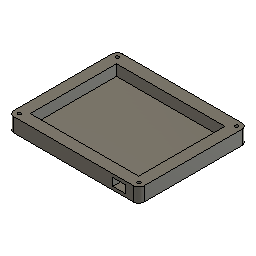
Final assemby 12 key hackpad (Autodesk Fusion 360 archive; units mm, degrees)
design "krish hackpad"
part number: 2026-03-11-19-54-52-839
Autodesk Fusion 360 part; units mm, degrees
sketch "hackpad base" plane through (0, 0, 0) normal (0, 1, 0) x (1, 0, 0)
  line L0 (0, 79.43) -> (0, 0)
  line L1 (0, 0) -> (99.82, 0)
  line L2 (99.82, 0) -> (99.82, 79.43)
  line L3 (99.82, 79.43) -> (0, 79.43)
  line L4 (-10, 90) -> (110, 90)
  line L5 (-10, -10) -> (-10, 90)
  line L6 (110, -10) -> (-10, -10)
  line L7 (110, 90) -> (110, -10)
  circle A0 centre (-5, -5) radius 1.45
  circle A1 centre (105, -5) radius 1.45
  circle A2 centre (105, 85) radius 1.45
  circle A3 centre (-5, 85) radius 1.45
extrude "Extrude1" add sketch "hackpad base" along normal blind 3 contours L0 L1 L2 L3 | L4 L5 L6 L7 makes body 1
extrude "Extrude2" add sketch "hackpad base" along normal blind 13 bodies 1
sketch "yes" plane through (0, 13, 0) normal (0, 1, 0) x (1, 0, 0)
  line L0 (4.775, 74.075) -> (17.775, 74.075)
  line L1 (4.775, 60.075) -> (17.775, 60.075)
  line L2 (4.275, 73.575) -> (4.275, 60.575)
  line L3 (18.275, 73.575) -> (18.275, 60.575)
  arc A0 (4.775, 74.075) -> (4.275, 73.575) centre (4.775, 73.575) ccw
  arc A1 (18.275, 73.575) -> (17.775, 74.075) centre (17.775, 73.575) ccw
  arc A2 (4.275, 60.575) -> (4.775, 60.075) centre (4.775, 60.575) ccw
  arc A3 (17.775, 60.075) -> (18.275, 60.575) centre (17.775, 60.575) ccw
  line L4 (23.825, 74.075) -> (36.825, 74.075)
  line L5 (23.825, 60.075) -> (36.825, 60.075)
  line L6 (23.325, 73.575) -> (23.325, 60.575)
  line L7 (37.325, 73.575) -> (37.325, 60.575)
  arc A4 (23.825, 74.075) -> (23.325, 73.575) centre (23.825, 73.575) ccw
  arc A5 (37.325, 73.575) -> (36.825, 74.075) centre (36.825, 73.575) ccw
  arc A6 (23.325, 60.575) -> (23.825, 60.075) centre (23.825, 60.575) ccw
  arc A7 (36.825, 60.075) -> (37.325, 60.575) centre (36.825, 60.575) ccw
  line L8 (42.875, 74.075) -> (55.875, 74.075)
  line L9 (42.875, 60.075) -> (55.875, 60.075)
  line L10 (42.375, 73.575) -> (42.375, 60.575)
  line L11 (56.375, 73.575) -> (56.375, 60.575)
  arc A8 (42.875, 74.075) -> (42.375, 73.575) centre (42.875, 73.575) ccw
  arc A9 (56.375, 73.575) -> (55.875, 74.075) centre (55.875, 73.575) ccw
  arc A10 (42.375, 60.575) -> (42.875, 60.075) centre (42.875, 60.575) ccw
  arc A11 (55.875, 60.075) -> (56.375, 60.575) centre (55.875, 60.575) ccw
  line L12 (61.925, 74.075) -> (74.925, 74.075)
  line L13 (61.925, 60.075) -> (74.925, 60.075)
  line L14 (61.425, 73.575) -> (61.425, 60.575)
  line L15 (75.425, 73.575) -> (75.425, 60.575)
  arc A12 (61.925, 74.075) -> (61.425, 73.575) centre (61.925, 73.575) ccw
  arc A13 (75.425, 73.575) -> (74.925, 74.075) centre (74.925, 73.575) ccw
  arc A14 (61.425, 60.575) -> (61.925, 60.075) centre (61.925, 60.575) ccw
  arc A15 (74.925, 60.075) -> (75.425, 60.575) centre (74.925, 60.575) ccw
  line L16 (4.775, 55.025) -> (17.775, 55.025)
  line L17 (4.775, 41.025) -> (17.775, 41.025)
  line L18 (4.275, 54.525) -> (4.275, 41.525)
  line L19 (18.275, 54.525) -> (18.275, 41.525)
  arc A16 (4.775, 55.025) -> (4.275, 54.525) centre (4.775, 54.525) ccw
  arc A17 (18.275, 54.525) -> (17.775, 55.025) centre (17.775, 54.525) ccw
  arc A18 (4.275, 41.525) -> (4.775, 41.025) centre (4.775, 41.525) ccw
  arc A19 (17.775, 41.025) -> (18.275, 41.525) centre (17.775, 41.525) ccw
  line L20 (23.825, 55.025) -> (36.825, 55.025)
  line L21 (23.825, 41.025) -> (36.825, 41.025)
  line L22 (23.325, 54.525) -> (23.325, 41.525)
  line L23 (37.325, 54.525) -> (37.325, 41.525)
  arc A20 (23.825, 55.025) -> (23.325, 54.525) centre (23.825, 54.525) ccw
  arc A21 (37.325, 54.525) -> (36.825, 55.025) centre (36.825, 54.525) ccw
  arc A22 (23.325, 41.525) -> (23.825, 41.025) centre (23.825, 41.525) ccw
  arc A23 (36.825, 41.025) -> (37.325, 41.525) centre (36.825, 41.525) ccw
  line L24 (42.875, 55.025) -> (55.875, 55.025)
  line L25 (42.875, 41.025) -> (55.875, 41.025)
  line L26 (42.375, 54.525) -> (42.375, 41.525)
  line L27 (56.375, 54.525) -> (56.375, 41.525)
  arc A24 (42.875, 55.025) -> (42.375, 54.525) centre (42.875, 54.525) ccw
  arc A25 (56.375, 54.525) -> (55.875, 55.025) centre (55.875, 54.525) ccw
  arc A26 (42.375, 41.525) -> (42.875, 41.025) centre (42.875, 41.525) ccw
  arc A27 (55.875, 41.025) -> (56.375, 41.525) centre (55.875, 41.525) ccw
  line L28 (61.925, 55.025) -> (74.925, 55.025)
  line L29 (61.925, 41.025) -> (74.925, 41.025)
  line L30 (61.425, 54.525) -> (61.425, 41.525)
  line L31 (75.425, 54.525) -> (75.425, 41.525)
  arc A28 (61.925, 55.025) -> (61.425, 54.525) centre (61.925, 54.525) ccw
  arc A29 (75.425, 54.525) -> (74.925, 55.025) centre (74.925, 54.525) ccw
  arc A30 (61.425, 41.525) -> (61.925, 41.025) centre (61.925, 41.525) ccw
  arc A31 (74.925, 41.025) -> (75.425, 41.525) centre (74.925, 41.525) ccw
  line L32 (4.775, 35.975) -> (17.775, 35.975)
  line L33 (4.775, 21.975) -> (17.775, 21.975)
  line L34 (4.275, 35.475) -> (4.275, 22.475)
  line L35 (18.275, 35.475) -> (18.275, 22.475)
  arc A32 (4.775, 35.975) -> (4.275, 35.475) centre (4.775, 35.475) ccw
  arc A33 (18.275, 35.475) -> (17.775, 35.975) centre (17.775, 35.475) ccw
  arc A34 (4.275, 22.475) -> (4.775, 21.975) centre (4.775, 22.475) ccw
  arc A35 (17.775, 21.975) -> (18.275, 22.475) centre (17.775, 22.475) ccw
  line L36 (23.825, 35.975) -> (36.825, 35.975)
  line L37 (23.825, 21.975) -> (36.825, 21.975)
  line L38 (23.325, 35.475) -> (23.325, 22.475)
  line L39 (37.325, 35.475) -> (37.325, 22.475)
  arc A36 (23.825, 35.975) -> (23.325, 35.475) centre (23.825, 35.475) ccw
  arc A37 (37.325, 35.475) -> (36.825, 35.975) centre (36.825, 35.475) ccw
  arc A38 (23.325, 22.475) -> (23.825, 21.975) centre (23.825, 22.475) ccw
  arc A39 (36.825, 21.975) -> (37.325, 22.475) centre (36.825, 22.475) ccw
  line L40 (42.875, 35.975) -> (55.875, 35.975)
  line L41 (42.875, 21.975) -> (55.875, 21.975)
  line L42 (42.375, 35.475) -> (42.375, 22.475)
  line L43 (56.375, 35.475) -> (56.375, 22.475)
  arc A40 (42.875, 35.975) -> (42.375, 35.475) centre (42.875, 35.475) ccw
  arc A41 (56.375, 35.475) -> (55.875, 35.975) centre (55.875, 35.475) ccw
  arc A42 (42.375, 22.475) -> (42.875, 21.975) centre (42.875, 22.475) ccw
  arc A43 (55.875, 21.975) -> (56.375, 22.475) centre (55.875, 22.475) ccw
  line L44 (61.925, 35.975) -> (74.925, 35.975)
  line L45 (61.925, 21.975) -> (74.925, 21.975)
  line L46 (61.425, 35.475) -> (61.425, 22.475)
  line L47 (75.425, 35.475) -> (75.425, 22.475)
  arc A44 (61.925, 35.975) -> (61.425, 35.475) centre (61.925, 35.475) ccw
  arc A45 (75.425, 35.475) -> (74.925, 35.975) centre (74.925, 35.475) ccw
  arc A46 (61.425, 22.475) -> (61.925, 21.975) centre (61.925, 22.475) ccw
  arc A47 (74.925, 21.975) -> (75.425, 22.475) centre (74.925, 22.475) ccw
  line L48 (4.775, 16.925) -> (17.775, 16.925)
  line L49 (4.775, 2.925) -> (17.775, 2.925)
  line L50 (4.275, 16.425) -> (4.275, 3.425)
  line L51 (18.275, 16.425) -> (18.275, 3.425)
  arc A48 (4.775, 16.925) -> (4.275, 16.425) centre (4.775, 16.425) ccw
  arc A49 (18.275, 16.425) -> (17.775, 16.925) centre (17.775, 16.425) ccw
  arc A50 (4.275, 3.425) -> (4.775, 2.925) centre (4.775, 3.425) ccw
  arc A51 (17.775, 2.925) -> (18.275, 3.425) centre (17.775, 3.425) ccw
  line L52 (23.825, 16.925) -> (36.825, 16.925)
  line L53 (23.825, 2.925) -> (36.825, 2.925)
  line L54 (23.325, 16.425) -> (23.325, 3.425)
  line L55 (37.325, 16.425) -> (37.325, 3.425)
  arc A52 (23.825, 16.925) -> (23.325, 16.425) centre (23.825, 16.425) ccw
  arc A53 (37.325, 16.425) -> (36.825, 16.925) centre (36.825, 16.425) ccw
  arc A54 (23.325, 3.425) -> (23.825, 2.925) centre (23.825, 3.425) ccw
  arc A55 (36.825, 2.925) -> (37.325, 3.425) centre (36.825, 3.425) ccw
  line L56 (42.875, 16.925) -> (55.875, 16.925)
  line L57 (42.875, 2.925) -> (55.875, 2.925)
  line L58 (42.375, 16.425) -> (42.375, 3.425)
  line L59 (56.375, 16.425) -> (56.375, 3.425)
  arc A56 (42.875, 16.925) -> (42.375, 16.425) centre (42.875, 16.425) ccw
  arc A57 (56.375, 16.425) -> (55.875, 16.925) centre (55.875, 16.425) ccw
  arc A58 (42.375, 3.425) -> (42.875, 2.925) centre (42.875, 3.425) ccw
  arc A59 (55.875, 2.925) -> (56.375, 3.425) centre (55.875, 3.425) ccw
  line L60 (61.925, 16.925) -> (74.925, 16.925)
  line L61 (61.925, 2.925) -> (74.925, 2.925)
  line L62 (61.425, 16.425) -> (61.425, 3.425)
  line L63 (75.425, 16.425) -> (75.425, 3.425)
  arc A60 (61.925, 16.925) -> (61.425, 16.425) centre (61.925, 16.425) ccw
  arc A61 (75.425, 16.425) -> (74.925, 16.925) centre (74.925, 16.425) ccw
  arc A62 (61.425, 3.425) -> (61.925, 2.925) centre (61.925, 3.425) ccw
  arc A63 (74.925, 2.925) -> (75.425, 3.425) centre (74.925, 3.425) ccw
  line L64 (1.75, 0.4) -> (77.95, 0.4)
  line L65 (1.75, 76.6) -> (77.95, 76.6)
  line L66 (1.75, 0.4) -> (1.75, 76.6)
  line L67 (77.95, 0.4) -> (77.95, 76.6)
sketch "Sketch3" plane through (0, 13, 0) normal (0, 1, 0) x (-1, 0, 0)
  circle A0 centre (5, 5) radius 1.45
  line L0 (0, -79.43) -> (-99.82, -79.43)
  line L1 (-99.82, -79.43) -> (-99.82, 0)
  line L2 (-99.82, 0) -> (0, 0)
  line L3 (0, 0) -> (0, -79.43)
  circle A1 centre (-105, 5) radius 1.45
  circle A2 centre (5, -85) radius 1.45
  circle A3 centre (-105, -85) radius 1.45
  line L4 (-110, -90) -> (10, -90)
  line L5 (10, -90) -> (10, 10)
  line L6 (10, 10) -> (-110, 10)
  line L7 (-110, 10) -> (-110, -90)
  line L8 (0, -79.43) -> (-99.82, -79.43)
  line L9 (-99.82, -79.43) -> (-99.82, 0)
  line L10 (-99.82, 0) -> (0, 0)
  line L11 (0, 0) -> (0, -79.43)
  constraint horizontal L8
  constraint vertical L9
  constraint horizontal L10
  constraint vertical L11
  constraint coincident L1.end L2.start
  constraint coincident L0.start L3.end
extrude "Extrude3" add sketch "Sketch3" along normal blind 3 separate body contours L0 L1 L2 L3 L8 L9 L10 L11 | L4 L5 L6 L7 makes body 2
extrude "Extrude4" cut sketch "yes" along normal blind 5 contours L0 L1 L2 L3 A0 A1 A2 A3 | L4 L5 L6 L7 A4 A5 A6 A7 | L8 L9 L10 L11 A8 A9 A10 A11 | L12 L13 L14 L15 A12 A13 A14 A15 | L16 L17 L18 L19 A16 A17 A18 A19 | L20 L21 L22 L23 A20 A21 A22 A23 | L24 L25 L26 L27 A24 A25 A26 A27 | L28 L29 L30 L31 A28 A29 A30 A31 | L32 L33 L34 L35 A32 A33 A34 A35 | L36 L37 L38 L39 A36 A37 A38 A39 | L40 L41 L42 L43 A40 A41 A42 A43 | L44 L45 L46 L47 A44 A45 A46 A47 | L48 L49 L50 L51 A48 A49 A50 A51 | L52 L53 L54 L55 A52 A53 A54 A55 | L56 L57 L58 L59 A56 A57 A58 A59 | L60 L61 L62 L63 A60 A61 A62 A63 bodies 2
fillet "Fillet1" radius 5 8 edges at (-10, 6.5, 10) (-10, 6.5, -90) (110, 6.5, -90) (110, 6.5, 10) (-10, 14.5, 10) (-10, 14.5, -90) (110, 14.5, -90) (110, 14.5, 10) on bodies 1 2
sketch "Sketch4" plane through (0, 16, 0) normal (0, 1, 0) x (-1, 0, 0)
  arc A0 (-105, 10) -> (-110, 5) centre (-105, 5) ccw
  line L0 (-110, 5) -> (-110, -85)
  arc A1 (-110, -85) -> (-105, -90) centre (-105, -85) ccw
  line L1 (-105, -90) -> (5, -90)
  arc A2 (5, -90) -> (10, -85) centre (5, -85) ccw
  line L2 (10, -85) -> (10, 5)
  arc A3 (10, 5) -> (5, 10) centre (5, 5) ccw
  line L3 (5, 10) -> (-105, 10)
  line L4 (-4.775, -35.975) -> (-17.775, -35.975)
  arc A4 (-18.275, -35.475) -> (-17.775, -35.975) centre (-17.775, -35.475) ccw
  line L5 (-18.275, -35.475) -> (-18.275, -22.475)
  arc A5 (-17.775, -21.975) -> (-18.275, -22.475) centre (-17.775, -22.475) ccw
  line L6 (-17.775, -21.975) -> (-4.775, -21.975)
  arc A6 (-4.275, -22.475) -> (-4.775, -21.975) centre (-4.775, -22.475) ccw
  line L7 (-4.275, -22.475) -> (-4.275, -35.475)
  arc A7 (-4.775, -35.975) -> (-4.275, -35.475) centre (-4.775, -35.475) ccw
  line L8 (-4.775, -74.075) -> (-17.775, -74.075)
  arc A8 (-18.275, -73.575) -> (-17.775, -74.075) centre (-17.775, -73.575) ccw
  line L9 (-18.275, -73.575) -> (-18.275, -60.575)
  arc A9 (-17.775, -60.075) -> (-18.275, -60.575) centre (-17.775, -60.575) ccw
  line L10 (-17.775, -60.075) -> (-4.775, -60.075)
  arc A10 (-4.275, -60.575) -> (-4.775, -60.075) centre (-4.775, -60.575) ccw
  line L11 (-4.275, -60.575) -> (-4.275, -73.575)
  arc A11 (-4.775, -74.075) -> (-4.275, -73.575) centre (-4.775, -73.575) ccw
  line L12 (-42.875, -55.025) -> (-55.875, -55.025)
  arc A12 (-56.375, -54.525) -> (-55.875, -55.025) centre (-55.875, -54.525) ccw
  line L13 (-56.375, -54.525) -> (-56.375, -41.525)
  arc A13 (-55.875, -41.025) -> (-56.375, -41.525) centre (-55.875, -41.525) ccw
  line L14 (-55.875, -41.025) -> (-42.875, -41.025)
  arc A14 (-42.375, -41.525) -> (-42.875, -41.025) centre (-42.875, -41.525) ccw
  line L15 (-42.375, -41.525) -> (-42.375, -54.525)
  arc A15 (-42.875, -55.025) -> (-42.375, -54.525) centre (-42.875, -54.525) ccw
  line L16 (-61.925, -16.925) -> (-74.925, -16.925)
  arc A16 (-75.425, -16.425) -> (-74.925, -16.925) centre (-74.925, -16.425) ccw
  line L17 (-75.425, -16.425) -> (-75.425, -3.425)
  arc A17 (-74.925, -2.925) -> (-75.425, -3.425) centre (-74.925, -3.425) ccw
  line L18 (-74.925, -2.925) -> (-61.925, -2.925)
  arc A18 (-61.425, -3.425) -> (-61.925, -2.925) centre (-61.925, -3.425) ccw
  line L19 (-61.425, -3.425) -> (-61.425, -16.425)
  arc A19 (-61.925, -16.925) -> (-61.425, -16.425) centre (-61.925, -16.425) ccw
  line L20 (-61.925, -35.975) -> (-74.925, -35.975)
  arc A20 (-75.425, -35.475) -> (-74.925, -35.975) centre (-74.925, -35.475) ccw
  line L21 (-75.425, -35.475) -> (-75.425, -22.475)
  arc A21 (-74.925, -21.975) -> (-75.425, -22.475) centre (-74.925, -22.475) ccw
  line L22 (-74.925, -21.975) -> (-61.925, -21.975)
  arc A22 (-61.425, -22.475) -> (-61.925, -21.975) centre (-61.925, -22.475) ccw
  line L23 (-61.425, -22.475) -> (-61.425, -35.475)
  arc A23 (-61.925, -35.975) -> (-61.425, -35.475) centre (-61.925, -35.475) ccw
  line L24 (-61.925, -74.075) -> (-74.925, -74.075)
  arc A24 (-75.425, -73.575) -> (-74.925, -74.075) centre (-74.925, -73.575) ccw
  line L25 (-75.425, -73.575) -> (-75.425, -60.575)
  arc A25 (-74.925, -60.075) -> (-75.425, -60.575) centre (-74.925, -60.575) ccw
  line L26 (-74.925, -60.075) -> (-61.925, -60.075)
  arc A26 (-61.425, -60.575) -> (-61.925, -60.075) centre (-61.925, -60.575) ccw
  line L27 (-61.425, -60.575) -> (-61.425, -73.575)
  arc A27 (-61.925, -74.075) -> (-61.425, -73.575) centre (-61.925, -73.575) ccw
  line L28 (-4.775, -55.025) -> (-17.775, -55.025)
  arc A28 (-18.275, -54.525) -> (-17.775, -55.025) centre (-17.775, -54.525) ccw
  line L29 (-18.275, -54.525) -> (-18.275, -41.525)
  arc A29 (-17.775, -41.025) -> (-18.275, -41.525) centre (-17.775, -41.525) ccw
  line L30 (-17.775, -41.025) -> (-4.775, -41.025)
  arc A30 (-4.275, -41.525) -> (-4.775, -41.025) centre (-4.775, -41.525) ccw
  line L31 (-4.275, -41.525) -> (-4.275, -54.525)
  arc A31 (-4.775, -55.025) -> (-4.275, -54.525) centre (-4.775, -54.525) ccw
  line L32 (-4.775, -16.925) -> (-17.775, -16.925)
  arc A32 (-18.275, -16.425) -> (-17.775, -16.925) centre (-17.775, -16.425) ccw
  line L33 (-18.275, -16.425) -> (-18.275, -3.425)
  arc A33 (-17.775, -2.925) -> (-18.275, -3.425) centre (-17.775, -3.425) ccw
  line L34 (-17.775, -2.925) -> (-4.775, -2.925)
  arc A34 (-4.275, -3.425) -> (-4.775, -2.925) centre (-4.775, -3.425) ccw
  line L35 (-4.275, -3.425) -> (-4.275, -16.425)
  arc A35 (-4.775, -16.925) -> (-4.275, -16.425) centre (-4.775, -16.425) ccw
  line L36 (-23.825, -35.975) -> (-36.825, -35.975)
  arc A36 (-37.325, -35.475) -> (-36.825, -35.975) centre (-36.825, -35.475) ccw
  line L37 (-37.325, -35.475) -> (-37.325, -22.475)
  arc A37 (-36.825, -21.975) -> (-37.325, -22.475) centre (-36.825, -22.475) ccw
  line L38 (-36.825, -21.975) -> (-23.825, -21.975)
  arc A38 (-23.325, -22.475) -> (-23.825, -21.975) centre (-23.825, -22.475) ccw
  line L39 (-23.325, -22.475) -> (-23.325, -35.475)
  arc A39 (-23.825, -35.975) -> (-23.325, -35.475) centre (-23.825, -35.475) ccw
  line L40 (-23.825, -74.075) -> (-36.825, -74.075)
  arc A40 (-37.325, -73.575) -> (-36.825, -74.075) centre (-36.825, -73.575) ccw
  line L41 (-37.325, -73.575) -> (-37.325, -60.575)
  arc A41 (-36.825, -60.075) -> (-37.325, -60.575) centre (-36.825, -60.575) ccw
  line L42 (-36.825, -60.075) -> (-23.825, -60.075)
  arc A42 (-23.325, -60.575) -> (-23.825, -60.075) centre (-23.825, -60.575) ccw
  line L43 (-23.325, -60.575) -> (-23.325, -73.575)
  arc A43 (-23.825, -74.075) -> (-23.325, -73.575) centre (-23.825, -73.575) ccw
  line L44 (-61.925, -55.025) -> (-74.925, -55.025)
  arc A44 (-75.425, -54.525) -> (-74.925, -55.025) centre (-74.925, -54.525) ccw
  line L45 (-75.425, -54.525) -> (-75.425, -41.525)
  arc A45 (-74.925, -41.025) -> (-75.425, -41.525) centre (-74.925, -41.525) ccw
  line L46 (-74.925, -41.025) -> (-61.925, -41.025)
  arc A46 (-61.425, -41.525) -> (-61.925, -41.025) centre (-61.925, -41.525) ccw
  line L47 (-61.425, -41.525) -> (-61.425, -54.525)
  arc A47 (-61.925, -55.025) -> (-61.425, -54.525) centre (-61.925, -54.525) ccw
  line L48 (-42.875, -16.925) -> (-55.875, -16.925)
  arc A48 (-56.375, -16.425) -> (-55.875, -16.925) centre (-55.875, -16.425) ccw
  line L49 (-56.375, -16.425) -> (-56.375, -3.425)
  arc A49 (-55.875, -2.925) -> (-56.375, -3.425) centre (-55.875, -3.425) ccw
  line L50 (-55.875, -2.925) -> (-42.875, -2.925)
  arc A50 (-42.375, -3.425) -> (-42.875, -2.925) centre (-42.875, -3.425) ccw
  line L51 (-42.375, -3.425) -> (-42.375, -16.425)
  arc A51 (-42.875, -16.925) -> (-42.375, -16.425) centre (-42.875, -16.425) ccw
  line L52 (-42.875, -35.975) -> (-55.875, -35.975)
  arc A52 (-56.375, -35.475) -> (-55.875, -35.975) centre (-55.875, -35.475) ccw
  line L53 (-56.375, -35.475) -> (-56.375, -22.475)
  arc A53 (-55.875, -21.975) -> (-56.375, -22.475) centre (-55.875, -22.475) ccw
  line L54 (-55.875, -21.975) -> (-42.875, -21.975)
  arc A54 (-42.375, -22.475) -> (-42.875, -21.975) centre (-42.875, -22.475) ccw
  line L55 (-42.375, -22.475) -> (-42.375, -35.475)
  arc A55 (-42.875, -35.975) -> (-42.375, -35.475) centre (-42.875, -35.475) ccw
  line L56 (-42.875, -74.075) -> (-55.875, -74.075)
  arc A56 (-56.375, -73.575) -> (-55.875, -74.075) centre (-55.875, -73.575) ccw
  line L57 (-56.375, -73.575) -> (-56.375, -60.575)
  arc A57 (-55.875, -60.075) -> (-56.375, -60.575) centre (-55.875, -60.575) ccw
  line L58 (-55.875, -60.075) -> (-42.875, -60.075)
  arc A58 (-42.375, -60.575) -> (-42.875, -60.075) centre (-42.875, -60.575) ccw
  line L59 (-42.375, -60.575) -> (-42.375, -73.575)
  arc A59 (-42.875, -74.075) -> (-42.375, -73.575) centre (-42.875, -73.575) ccw
  line L60 (-23.825, -55.025) -> (-36.825, -55.025)
  arc A60 (-37.325, -54.525) -> (-36.825, -55.025) centre (-36.825, -54.525) ccw
  line L61 (-37.325, -54.525) -> (-37.325, -41.525)
  arc A61 (-36.825, -41.025) -> (-37.325, -41.525) centre (-36.825, -41.525) ccw
  line L62 (-36.825, -41.025) -> (-23.825, -41.025)
  arc A62 (-23.325, -41.525) -> (-23.825, -41.025) centre (-23.825, -41.525) ccw
  line L63 (-23.325, -41.525) -> (-23.325, -54.525)
  arc A63 (-23.825, -55.025) -> (-23.325, -54.525) centre (-23.825, -54.525) ccw
  line L64 (-23.825, -16.925) -> (-36.825, -16.925)
  arc A64 (-37.325, -16.425) -> (-36.825, -16.925) centre (-36.825, -16.425) ccw
  line L65 (-37.325, -16.425) -> (-37.325, -3.425)
  arc A65 (-36.825, -2.925) -> (-37.325, -3.425) centre (-36.825, -3.425) ccw
  line L66 (-36.825, -2.925) -> (-23.825, -2.925)
  arc A66 (-23.325, -3.425) -> (-23.825, -2.925) centre (-23.825, -3.425) ccw
  line L67 (-23.325, -3.425) -> (-23.325, -16.425)
  arc A67 (-23.825, -16.925) -> (-23.325, -16.425) centre (-23.825, -16.425) ccw
  circle A68 centre (5, -85) radius 1.45
  circle A69 centre (-105, 5) radius 1.45
  circle A70 centre (5, 5) radius 1.45
  circle A71 centre (-105, -85) radius 1.45
  line L68 (-94.275, -68.595) -> (-82.275, -68.595)
  line L69 (-82.275, -68.595) -> (-82.275, -39.095)
  line L70 (-82.275, -39.095) -> (-94.275, -39.095)
  line L71 (-94.275, -39.095) -> (-94.275, -68.595)
  line L72 (-99.82, -79.43) -> (0, -79.43)
  line L73 (-77.95, -0.4) -> (-77.95, -76.6)
  dimension "d11" = 12
  dimension "d12" = 29.5
  dimension "d13" = 10.835
  dimension "d14" = 4.325
  constraint horizontal L68
  constraint vertical L69
  constraint horizontal L70
  constraint vertical L71
  measures "d11" distance of L68.start L68.end
  measures "d12" distance of L68.start L70.end
  measures "d13" distance of L68 L72
  measures "d14" distance of L69 L73
extrude "Extrude5" cut sketch "Sketch4" against normal blind 5 contours L68 L69 L70 L71 bodies 2
sketch "Sketch5" plane through (0, 0, 10) normal (0, 0, 1) x (1, 0, 0)
  line L0 (105, 0) -> (105, 13)
  line L1 (105, 13) -> (-5, 13)
  line L2 (-5, 13) -> (-5, 0)
  line L3 (-5, 0) -> (105, 0)
  line L4 (97.35, 2.9398) -> (86, 2.9398)
  line L5 (86, 2.9398) -> (86, 10)
  line L6 (86, 10) -> (97.35, 10)
  line L7 (97.35, 10) -> (97.35, 2.9398)
  constraint horizontal L4
  constraint vertical L5
  constraint horizontal L6
  constraint vertical L7
extrude "Extrude6" cut sketch "Sketch5" against normal blind 10 contours L4 L5 L6 L7 bodies 1
hidden bodies 2
